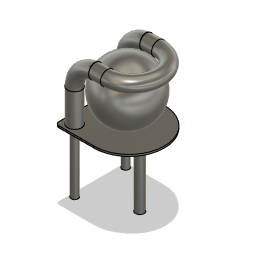
Stern Newton Ball Assembly (Autodesk Fusion 360 design; units mm, degrees)
part number: 535-9523-00
part number: 535-9522-00
Autodesk Fusion 360 part; units mm, degrees
note: some values were not read from the file. Chosen so that the rebuilt part matches the saved one: which face or edge a step refers to.
sketch "Sketch1" plane through (0, 0, 0) normal (0, 1, 0) x (1, 0, 0) in component "Base"
  line L0 (0, 1.5875) -> (31.75, 1.5875)
  line L1 (31.75, 1.5875) -> (31.75, 17.4625)
  line L2 (31.75, 17.4625) -> (0, 17.4625)
  line L3 (0, 17.4625) -> (0, 1.5875)
  arc A0 (0, 1.5875) -> (1.5875, 0) centre (1.5875, 1.5875) ccw
  arc A1 (30.1625, 0) -> (31.75, 1.5875) centre (30.1625, 1.5875) ccw
  line L4 (1.5875, 0) -> (30.1625, 0)
  circle A2 centre (4.3656, 4.3656) radius 2.1828
  circle A3 centre (27.3844, 4.3656) radius 2.1828
  arc A4 (31.75, 17.4625) -> (0, 17.4625) centre (15.875, 17.4625) ccw
  point P0 (1.5875, 0)
  point P1 (30.1625, 0)
  point P2 (27.3844, 4.3656)
  point P3 (4.3656, 4.3656)
  dimension "d1" = 4.3656
  dimension "d2" = 4.3656
  constraint horizontal L0
  constraint vertical L1
  constraint horizontal L2
  constraint vertical L3
  constraint tangent L3 A0
  constraint coincident P0 A0.end
  constraint tangent L1 A1
  constraint coincident P1 A1.start
  constraint tangent A1 L4
  constraint coincident P3 A2.centre
  constraint coincident P2 A3.centre
  constraint tangent L3 A4
  measures "d1" diameter of A2
  measures "d2" diameter of A3
extrude "Face1" add sketch "Sketch1" sketch "Sketch1" sketch "Sketch1" along normal blind 0.7937 contours L2 A4 of sketch 2 contours L0 L1 L2 L3 | L2 A4 of sketch 3 makes body 1 in component "Base"
sketch "Sketch2" plane through (0, 0, 0) normal (0, 0, 1) x (1, 0, 0) in component "Base"
  line L0 (1.5875, 0) -> (30.1625, 0)
ref_plane "WorkPlane1" through (15.875, -30.1625, -16.6687) normal (0, -1, 0) x (-1, 0, 0) in component "Base"
sketch "Sketch3" plane through (15.875, -30.1625, -16.6687) normal (0, -1, 0) x (1, 0, 0) in component "Base"
  circle A0 centre (0, 16.6687) radius 1.9844
  point P0 (0, 16.6687)
  dimension "d6" = 3.9688
  constraint coincident P0 A0.centre
  measures "d6" diameter of A0
extrude "Extrude1" add sketch "Sketch3" against normal blind 30.1625 bodies 1 in component "Base"
move_face "MoveFace1" to x (1, 0, 0) y (0, 1, 0) z (0, 0, 1) at (0, 0, -22.225) 2 faces at (14.2397, -10.0542, -1.1241) (16.4435, -30.1625, -0.469) on bodies 1 in component "Base"
sketch "Sketch1 (2)" plane through (0, 0, 0) normal (1, 0, 0) x (0, 0, -1) in component "Lock Down"
  line L0 (0, 0) -> (0, 14.6844)
  arc A0 (9.525, 25.4) -> (0, 14.6844) centre (10.79, 14.6844) ccw
  line L1 (9.525, 25.4) -> (21.159, 25.4412)
  dimension "d12" = 14.6844
  constraint coincident L0.start origin
  constraint vertical L0
  constraint tangent L0 A0
  measures "d12" distance of L0.start L0.end
sketch "Sketch2 (2)" plane through (0, 0, 0) normal (0, 1, 0) x (1, 0, 0) in component "Lock Down"
  circle A0 centre (0, 0) radius 3.175
  dimension "d14" = 6.35
  constraint coincident A0.centre origin
  measures "d14" diameter of A0
sweep "Sweep1" add profiles "Sketch2 (2)" path "Sketch1 (2)" along L0 A0 L1 section 1 separate body makes body 2 in component "Lock Down"
sketch "Sketch3 (2)" plane through (0, 0, 0) normal (0, -1, 0) x (1, 0, 0) in component "Lock Down"
  circle A0 centre (0, 0) radius 3.175
  circle A1 centre (0, 0) radius 1.5875
  dimension "d21" = 3.175
  constraint coincident A0.centre A1.centre
  measures "d21" diameter of A1
extrude "Extrude1'" add sketch "Sketch3 (2)" along normal blind 28.575 contours A1 bodies 2 in component "Lock Down"
move_face "OffsetFaces1" offset -6.35 1 faces at (0.8826, 24.5008, -21.1623) on bodies 2 in component "Lock Down"
copy_body "CopyPasteBodies1" bodies 2 makes body 3 in component "Lock Down"
move_body "Move1" bodies 3 to x (1, 0, 0) y (0, 1, 0) z (0, 0, 1) at (18.1504, 18.2293, 0) in component "Lock Down"
move_body "Move2" bodies 3 to x (1, 0, 0) y (0, 1, 0) z (0, 0, 1) at (4.8684, -18.2293, 0) in component "Lock Down"
ref_plane "WorkPlane1" through (23.0187, 25.3853, -5.3751) normal (0, -0.999994, -0.003537) x (1, 0, 0) in component "Lock Down"
sketch "Sketch4" plane through (23.0187, 25.3853, -5.3751) normal (0, -0.999994, -0.003537) x (1, 0, 0) in component "Lock Down"
  line L0 (-26.1937, -9.4339) -> (-19.8437, -9.4339)
  line L1 (-3.175, -9.4339) -> (3.175, -9.4339)
  arc A0 (-23.0187, -9.4339) -> (0, -9.4339) centre (-11.5094, -9.4339) ccw
  constraint midpoint L0 A0.start
  constraint midpoint L1 A0.end
sweep "Sweep2" add 1 faces at (23.475, 24.7577, -14.8114) path "Sketch4" along A0 on bodies 3 bodies 3 2 in component "Lock Down"
sphere "SpherePrimitive1" add diameter 26.9875 placed x (1, 0, 0) y (0, 0, -1) z (0, 1, 0) at (73.9443, 0, -14.933) separate body makes body 4 in component "Ball"
move_body "MoveFace1'" bodies 4 to x (1, 0, 0) y (0, 1, 0) z (0, 0, 1) at (-57.9438, 0, 0) on bodies 4 in component "Ball"
move_body "MoveFace2" bodies 4 to x (1, 0, 0) y (0, 1, 0) z (0, 0, 1) at (0, 12.7, 0) on bodies 4 in component "Ball"
move_body "MoveFace3" bodies 4 to x (1, 0, 0) y (0, 1, 0) z (0, 0, 1) at (0, 0.7937, 0) on bodies 4 in component "Ball"
move_body "MoveFace4" bodies 4 to x (1, 0, 0) y (0, 1, 0) z (0, 0, 1) at (0, 0.7937, 0) on bodies 4 in component "Ball"
move_body "MoveFace5" bodies 4 to x (1, 0, 0) y (0, 1, 0) z (0, 0, 1) at (0, 0, -6.35) on bodies 4 in component "Ball"
move_body "MoveFace6" bodies 4 to x (1, 0, 0) y (0, 1, 0) z (0, 0, 1) at (0, 0, 1.5875) on bodies 4 in component "Ball"
move_body "MoveFace7" bodies 4 to x (1, 0, 0) y (0, 1, 0) z (0, 0, 1) at (0, 0, 3.175) on bodies 4 in component "Ball"
component "Base" placed x (1, 0, 0) y (0, 1, 0) z (0, 0, 1) at (0, 0, 0)
component "Lock Down" placed x (1, 0, 0) y (0, 1, 0) z (0, 0, 1) at (4.3656, 0.7937, -4.3656)
component "Ball" placed x (1, 0, 0) y (0, 1, 0) z (0, 0, 1) at (-0.1984, 0, 0)
equation "d1 = ( 11 / 64 ) * 1 in"
equation "d2 = ( 11 / 64 ) * 1 in"
equation "d3 = ( 1 / 32 ) * 1 in"
equation "d5 = 1 3/16\""
equation "d6 = ( 5 / 32 ) * 1 in"
equation "d7 = -1 3/16\""
equation "d11 = ( -7 / 8 ) * 1 in"
equation "d12 = ( 37 / 64 ) * 1 in"
equation "d14 = ( 1 / 4 ) * 1 in"
equation "d21 = ( 1 / 8 ) * 1 in"
equation "d22 = 1 1/8\""
equation "d32 = 1 1/16\""
equation "d33 = -2 9/32\""
equation "d40 = ( 1 / 32 ) * 1 in"
equation "d43 = ( 1 / 32 ) * 1 in"
equation "d47 = ( -1 / 4 ) * 1 in"
equation "d50 = ( 1 / 16 ) * 1 in"
equation "d53 = ( 2 / 16 ) * 1 in"
